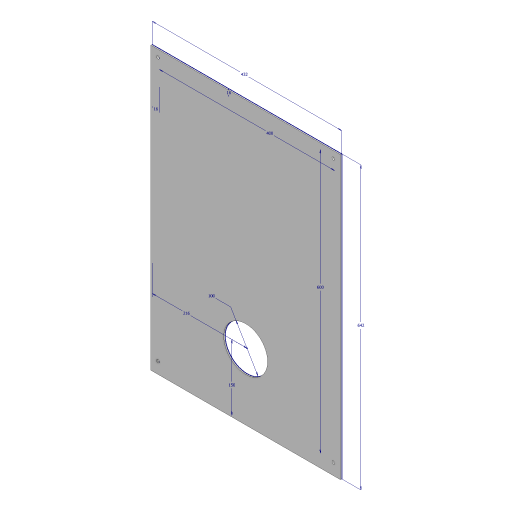
# Autodesk Inventor part: top-ventilation-hole-100mm
Saved by Autodesk Inventor 2023 (Build 270158000, 158)
## iProperties
Created: 2024-06-07
Part Number: top-ventilation-hole-100mm
Material: Generic
Document SubType Name: Modeling
Designer: nvladi
Density: 1 g/cm^3
Appearance: Default
Author: nvladi
Autodesk Inventor part; units mm, degrees
ref_plane "YZ Plane" through (0, 0, 0) normal (1, 0, 0) x (0, 1, 0)
ref_plane "XZ Plane" through (0, 0, 0) normal (0, 1, 0) x (-1, 0, 0)
ref_plane "XY Plane" through (0, 0, 0) normal (0, 0, 1) x (1, 0, 0)
sketch "Sketch1" plane through (0, 0, 0) normal (0, 0, 1) x (1, 0, 0)
  line L0 (0, 0) -> (432, 0)
  line L1 (432, 0) -> (432, 642)
  line L2 (432, 642) -> (0, 642)
  line L3 (0, 642) -> (0, 0)
  line L4 (16, 626) -> (16, 26) construction
  line L5 (416, 626) -> (416, 26) construction
  line L6 (16, 626) -> (416, 626) construction
  line L7 (16, 26) -> (416, 26) construction
  circle A0 centre (216, 150) radius 50
  dimension "d0" = 432
  dimension "d1" = 642
  dimension "d2" = 600
  dimension "d3" = 400
  dimension "d4" = 16
  dimension "d5" = 16
  dimension "d6" = 100
  dimension "d7" = 150
  dimension "d8" = 216
  constraints: 16 end point, 4 coincident, 3 parallel, 2 horizontal, 2 vertical, 1 centre point, 1 perpendicular
  measures "d0" distance of L2.end L1.end
  measures "d1" distance of L1.end L0.end
  measures "d2" distance between parallel lines of L7 L6
  measures "d3" distance between parallel lines of L5 L4
  measures "d4" distance between parallel lines of L3 L4
  measures "d5" distance between parallel lines of L6 L2
  measures "d6" diameter of A0
  measures "d7" distance from line of L0 A0.centre
  measures "d8" distance from line of L3 A0.centre
extrude "Extrusion1" add sketch "Sketch1" along normal blind 3
hole "Hole1" at (16, 626, 0) at (416, 626, 0) at (416, 26, 0) at (16, 26, 0) direction (0, 0, 1) diameter 6.4 end through all
body "Solid1"
